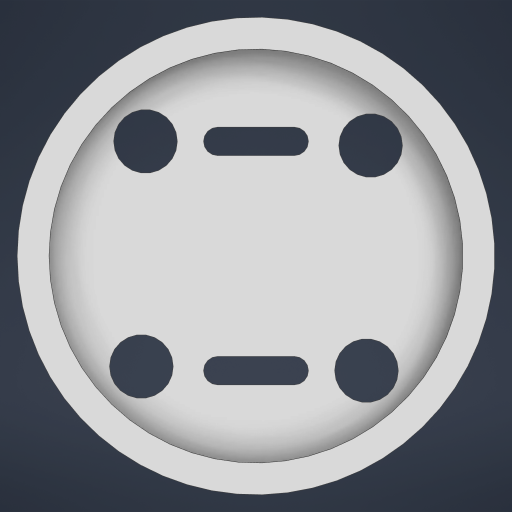
# Autodesk Inventor part: case_top
Saved by Autodesk Inventor 2023 (Build 270158000, 158)
## iProperties
Created: 2022-11-18
Part Number: case_top
Material: Generic
Document SubType Name: Modeling
Designer: washington
Density: 1 g/cm^3
Appearance: Default
Author: washington
Autodesk Inventor part; units mm, degrees
ref_plane "YZ Plane" through (0, 0, 0) normal (1, 0, 0) x (0, 1, 0)
ref_plane "XZ Plane" through (0, 0, 0) normal (0, 1, 0) x (-1, 0, 0)
ref_plane "XY Plane" through (0, 0, 0) normal (0, 0, 1) x (1, 0, 0)
sketch "Sketch1" plane through (0, 0, 0) normal (0, 1, 0) x (-1, 0, 0)
  circle A0 centre (0, 0) radius 32.5
  circle A1 centre (0, 0) radius 25
  circle A2 centre (17.3494, -18) radius 5
  circle A3 centre (18, 17.3494) radius 5
  circle A4 centre (-17.3494, 18) radius 5
  circle A5 centre (-18, -17.3494) radius 5
  line L0 (6, -18) -> (-6, -18) construction
  line L1 (6, -15.7639) -> (-6, -15.7639)
  line L2 (-6, -20.2361) -> (6, -20.2361)
  arc A6 (6, -20.2361) -> (6, -15.7639) centre (6, -18) ccw
  arc A7 (-6, -15.7639) -> (-6, -20.2361) centre (-6, -18) ccw
  line L3 (-25, 0) -> (25, 0) construction
  line L4 (6, 15.7639) -> (-6, 15.7639)
  line L5 (-6, 20.2361) -> (6, 20.2361)
  arc A8 (6, 15.7639) -> (6, 20.2361) centre (6, 18) ccw
  arc A9 (-6, 20.2361) -> (-6, 15.7639) centre (-6, 18) ccw
  circle A10 centre (0, 0) radius 37.5
  point P0 (0, -18)
  dimension "d0" = 65
  dimension "d1" = 50
  dimension "d2" = 10
  dimension "d5" = 360
  dimension "d7" = 35.3494
  dimension "d11" = 17.3494
  dimension "d12" = 11.3493
  dimension "d16" = 18
  dimension "d17" = 2.2361
  dimension "d18" = 18
  dimension "d19" = 75
  constraints: 14 end point, 11 centre point, 11 point on circle, 6 symmetric about line, 4 tangent, 3 coincident, 2 horizontal, 1 midpoint, 1 parallel, 11 other
  measures "d0" diameter of A0
  measures "d1" diameter of A1
  measures "d2" diameter of A2
  measures "d7" horizontal distance of A4.centre A3.centre
  measures "d11" distance of A2.centre point (0, -18)
  measures "d12" distance of A2.centre L0.start
  measures "d16" distance of point (0, -18) point (0, 0)
  measures "d17" radius of A6
  measures "d18" distance between parallel lines of L3 L0
  measures "d19" diameter of A10
extrude "Extrusion1" add sketch "Sketch1" against normal blind 10 contours A0 | A1 A2 A5 A4 A3
extrude "Extrusion2" add sketch "Sketch1" along normal blind 10 and the other way blind 10 contours A10
body "Solid1"
